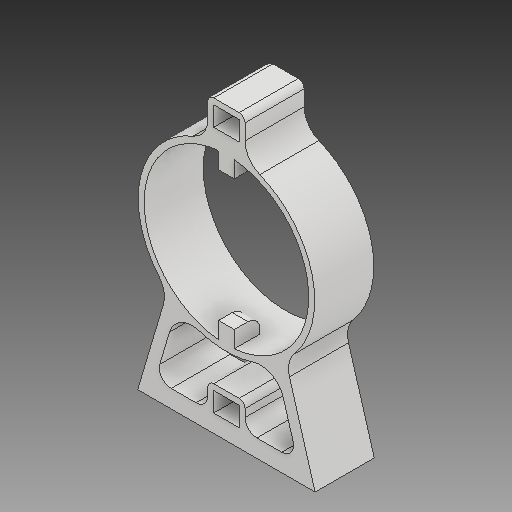
# Autodesk Inventor part: Motor Reversed Mount
Saved by Autodesk Inventor 2018 (Build 220112000, 112)
## iProperties
Created: 2018-01-25
Part Number: Motor Reversed Mount
Material: ABS Plastic
Document SubType Name: Modeling
Designer: Moochster
Density: 1.06 g/cm^3
Appearance: Smooth - White
Mass: 3.13217 g
Surface Area: 39.5501 cm^2
Volume: 2.95488 cm^3
Author: Moochster
Autodesk Inventor part; units mm, degrees
ref_plane "YZ Plane" through (0, 0, 0) normal (1, 0, 0) x (0, 1, 0)
ref_plane "XZ Plane" through (0, 0, 0) normal (0, 1, 0) x (-1, 0, 0)
ref_plane "XY Plane" through (0, 0, 0) normal (0, 0, 1) x (1, 0, 0)
sketch "Sketch1" plane through (0, 0, 0) normal (0, 0, 1) x (1, 0, 0)
  circle A0 centre (0, 0) radius 13.92
  circle A1 centre (0, 0) radius 14.92
  line L0 (-10, -11.0728) -> (-15, -28)
  line L1 (-15, -28) -> (15, -28)
  line L2 (15, -28) -> (10, -11.0728)
  line L3 (8.3051, -12.3948) -> (12.0284, -25)
  line L4 (12.0284, -25) -> (-12.0284, -25)
  line L5 (-12.0284, -25) -> (-8.3051, -12.3948)
  line L6 (-2, -22) -> (2, -22) construction
  line L7 (2, -22) -> (2, -25) construction
  line L8 (2, -25) -> (-2, -25) construction
  line L9 (-2, -25) -> (-2, -22) construction
  line L10 (2.15, -21.7) -> (-2.15, -21.7)
  line L11 (-2.15, -21.7) -> (-2.15, -25)
  line L12 (-2.15, -25) -> (2.15, -25) construction
  line L13 (2.15, -25) -> (2.15, -25)
  line L14 (2.15, -25) -> (2.15, -21.7)
  line L15 (-2.15, -25) -> (-2.15, -25)
  line L16 (-3.15, -25) -> (-3.15, -20.7)
  line L17 (-3.15, -20.7) -> (3.15, -20.7)
  line L18 (3.15, -20.7) -> (3.15, -25)
  line L19 (-1.48, 13.8411) -> (-1.48, 10.8811) construction
  line L20 (-1.48, 10.8811) -> (1.48, 10.8811) construction
  line L21 (1.48, 10.8811) -> (1.48, 13.8411) construction
  line L22 (1.33, 13.8563) -> (1.33, 11.0311)
  line L23 (1.33, 11.0311) -> (-1.33, 11.0311)
  line L24 (-1.33, 11.0311) -> (-1.33, 13.8563)
  line L25 (-1.33, -13.8563) -> (-1.33, -11.0311)
  line L26 (-1.33, -11.0311) -> (1.33, -11.0311)
  line L27 (1.33, -11.0311) -> (1.33, -13.8563)
  line L28 (2, 20) -> (-2, 20) construction
  line L29 (-2, 20) -> (-2, 17) construction
  line L30 (-2, 17) -> (2, 17) construction
  line L31 (2, 17) -> (2, 20) construction
  line L32 (-2.15, 16.85) -> (-2.15, 20.15)
  line L33 (-2.15, 20.15) -> (2.15, 20.15)
  line L34 (2.15, 20.15) -> (2.15, 16.85)
  line L35 (2.15, 16.85) -> (-2.15, 16.85)
  line L36 (3.15, 14.5837) -> (3.15, 21.15)
  line L37 (3.15, 21.15) -> (-3.15, 21.15)
  line L38 (-3.15, 21.15) -> (-3.15, 14.5837)
  point P0 (0, -22)
  point P1 (0, 10.8811)
  point P2 (0, 20)
  dimension "d0" = 27.84
  dimension "d1" = 1
  dimension "d2" = 3
  dimension "d3" = 2
  dimension "d4" = 2
  dimension "d5" = 28
  dimension "d6" = 30
  dimension "d7" = 20
  dimension "d10" = 3
  dimension "d11" = 4
  dimension "d12" = 3
  dimension "d13" = 0.3
  dimension "d14" = 0.15
  dimension "d15" = 0.15
  dimension "d16" = 1
  dimension "d17" = 1
  dimension "d18" = 1
  dimension "d22" = 2.96
  dimension "d23" = 2.96
  dimension "d24" = 0.15
  dimension "d25" = 0.15
  dimension "d26" = 0.15
  dimension "d30" = 3
  dimension "d31" = 4
  dimension "d32" = 17
  dimension "d33" = 0.15
  dimension "d34" = 1
  dimension "d35" = 1
  dimension "d36" = 1
  constraints: 78 end point, 13 parallel, 13 perpendicular, 12 point on circle, 5 vertical, 5 vertical alignment, 4 horizontal, 4 point on line, 3 midpoint, 2 centre point, 2 coincident, 2 equal length, 1 collinear, 1 horizontal alignment, 3 other
  measures "d0" diameter of A0
  measures "d1" radial gap between concentric circles of A0 A1
  measures "d2" distance between parallel lines of L1 L4
  measures "d3" distance between parallel lines of L0 L5
  measures "d4" distance between parallel lines of L2 L3
  measures "d5" distance from line of point (0, 0) L1
  measures "d6" distance of L0.end L1.end
  measures "d7" distance of L0.start L2.end
  measures "d10" distance of L6.end L7.end
  measures "d11" distance of L7.end L8.end
  measures "d12" distance between parallel lines of L1 L8
  measures "d13" distance between parallel lines of L10 L6
  measures "d14" distance between parallel lines of L7 L14
  measures "d15" distance between parallel lines of L9 L11
  measures "d16" distance between parallel lines of L17 L10
  measures "d17" distance between parallel lines of L14 L18
  measures "d18" distance between parallel lines of L16 L11
  measures "d22" distance of L20.end L21.end
  measures "d23" distance of L19.end L20.end
  measures "d24" distance between parallel lines of L21 L22
  measures "d25" distance between parallel lines of L20 L23
  measures "d26" distance between parallel lines of L19 L24
  measures "d30" distance of L28.end L29.end
  measures "d31" distance of L28.start L28.end
  measures "d32" distance from line of point (0, 0) L30
  measures "d33" distance between parallel lines of L29 L32
  measures "d34" distance between parallel lines of L32 L38
  measures "d35" distance between parallel lines of L36 L34
  measures "d36" distance between parallel lines of L37 L33
extrude "Extrusion1" add sketch "Sketch1" along normal blind 10 contours A1 | A1 L38 L37 L36 | L2 L1 L0 A1 L5 L4 L3 | L4 L14 L10 L11 L16 L17 L18
fillet "Fillet1" radius 4 6 edges at (10, -11.0728, 5) (-10, -11.0728, 5) (-8.3051, -12.3948, 5) (8.3051, -12.3948, 5) (3.15, 14.5837, 5) (-3.15, 14.5837, 5)
fillet "Fillet1" radius 2 4 edges at (-12.0284, -25, 5) (12.0284, -25, 5) (3.15, -25, 5) (-3.15, -25, 5)
fillet "Fillet1" radius 1 4 edges at (-3.15, -20.7, 5) (3.15, -20.7, 5) (3.15, 21.15, 5) (-3.15, 21.15, 5)
extrude "Extrusion2" add sketch "Sketch1" along normal blind 4.3 contours L22 L23 L24 A0 | A0 L25 L26 L27
fillet "Fillet2" radius 2 2 edges at (0, -11.0311, 4.3) (0, 11.0311, 4.3)
body "Solid1"
